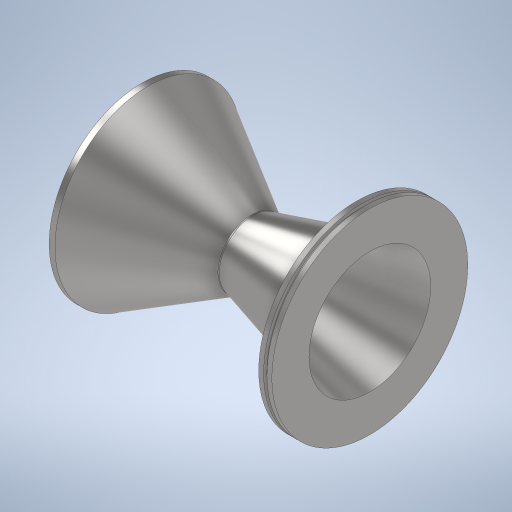
# Autodesk Inventor part: stainless steel final nozzle
Saved by Autodesk Inventor 2023 (Build 270158000, 158)
## iProperties
Created: 2022-09-19
Part Number: stainless steel final nozzle
Material: Stainless Steel
Document SubType Name: Modeling
Designer: station
Density: 8 g/cm^3
Appearance: Semi-Polished
Author: station
Autodesk Inventor part; units mm, degrees
ref_plane "YZ Plane" through (0, 0, 0) normal (1, 0, 0) x (0, 1, 0)
ref_plane "XZ Plane" through (0, 0, 0) normal (0, 1, 0) x (-1, 0, 0)
ref_plane "XY Plane" through (0, 0, 0) normal (0, 0, 1) x (1, 0, 0)
sketch "Sketch1" plane through (0, 0, 0) normal (0, 0, 1) x (1, 0, 0)
  line L0 (254.7886, 18.124) -> (254.7886, 0) construction
  line L1 (192, 54.375) -> (254.7886, 18.124)
  line L2 (0, 0) -> (487.78, 0)
  line L3 (254.7886, 18.124) -> (256.7886, 18.124)
  line L4 (256.7886, 18.124) -> (327.1228, 36.97)
  line L5 (327.1228, 36.97) -> (327.1228, 0)
  line L6 (327.1228, 40.0758) -> (255.8936, 20.258)
  line L7 (255.8936, 20.258) -> (255.0924, 20.258)
  line L8 (255.0924, 20.258) -> (192.3194, 56.5)
  line L9 (327.1228, 36.97) -> (327.1228, 40.0758)
  line L10 (192, 54.375) -> (191.7835, 54.5)
  line L11 (0, 0) -> (0, 54.5)
  line L12 (0, 54.5) -> (274.8621, 54.5) construction
  line L13 (191.7835, 54.5) -> (188.7835, 54.5)
  line L14 (188.7835, 54.5) -> (188.7835, 56.5)
  line L15 (188.7835, 56.5) -> (192.3194, 56.5)
  line L16 (327.1228, 0) -> (327.1228, 59.5)
  line L17 (327.1228, 59.5) -> (323.1228, 59.5)
  line L18 (323.1228, 59.5) -> (319.1228, 59.5)
  line L19 (319.1228, 59.5) -> (319.1228, 37.85)
  point P0 (322.4487, 38.7754)
  point P1 (191.9595, 55.4142)
  point P2 (188.9595, 55.4)
  point P3 (323.1228, 38.9629)
  dimension "d2" = 18.124
  dimension "d4" = 30
  dimension "d5" = 18.124
  dimension "d6" = 2
  dimension "d7" = 15
  dimension "d8" = 36.97
  dimension "d9" = 2
  dimension "d19" = 54.5
  dimension "d20" = 3
  dimension "d21" = 2
  dimension "d22" = 59.5
  dimension "d23" = 4
  dimension "d24" = 4
  constraints: 40 end point, 7 point on line, 6 perpendicular, 3 horizontal, 2 vertical, 1 parallel
  measures "d2" distance of L0.start L0.end
  measures "d4" angle of L2 L1
  measures "d5" distance from line of L2 L0.start
  measures "d6" distance of L0.start L3.end
  measures "d7" angle of L2 L4
  measures "d8" distance of L4.end L5.end
  measures "d9" distance between parallel lines of L1 L8
  measures "d19" distance of L2.start L11.end
  measures "d20" distance of L10.end L13.end
  measures "d21" distance of L13.end L14.end
  measures "d22" distance of L5.end L16.end
  measures "d23" distance of L16.end L17.end
  measures "d24" distance of L17.end L18.end
revolve "Revolution1" add sketch "Sketch1" angle 360 about axis through (0, 0, 0) along (1, 0, 0)
sketch "Sketch2" plane through (0, 0, 0) normal (0, 0, 1) x (1, 0, 0)
  line L0 (319.1228, -59.5) -> (319.1228, 59.5) projected
  line L1 (319.1228, 59.5) -> (322.1228, 59.5)
  line L2 (319.1228, 59.5) -> (327.1228, 59.5) projected
  line L3 (322.1228, 59.5) -> (324.1228, 59.5)
  line L4 (324.1228, 59.5) -> (324.1228, 57.5)
  line L5 (324.1228, 57.5) -> (322.1228, 57.5)
  line L6 (322.1228, 57.5) -> (322.1228, 59.5)
  line L7 (-65.4246, 0) -> (392.5474, 0) projected
  point P0 (0, 0)
  dimension "d25" = 3
  dimension "d26" = 2
  dimension "d27" = 2
  constraints: 10 end point, 2 parallel, 1 horizontal, 1 perpendicular, 1 point on line
  measures "d25" distance of L0.end L1.end
  measures "d26" distance of L4.end L5.end
  measures "d27" distance of L3.end L4.end
revolve "Revolution2" cut sketch "Sketch2" angle 360 about axis through (-10, 0, 0) along (1, 0, 0)
body "Solid1"
